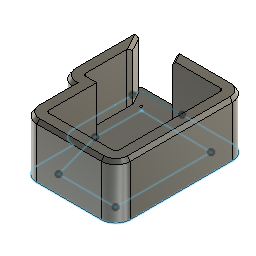
isopad-case-bigswitch v6 (Autodesk Fusion 360 design; units mm, degrees)
Autodesk Fusion 360 part; units mm, degrees
note: some values were not read from the file. Set by a fixed rule: which sketch regions a step uses.
(part 1 of 3)
sketch "isopad-Edge_Cuts" plane through (0, 0, 0) normal (0, 0, 1) x (1, 0, 0)
  line L0 (124.655, -116.632) -> (124.654, -116.632)
  line L1 (150.738, -76.6321) -> (150.718, -116.273)
  line L2 (125.094, -116.865) -> (125.093, -116.865)
  line L3 (150.127, -116.867) -> (150.124, -116.867)
  line L4 (150.128, -116.867) -> (150.127, -116.867)
  line L5 (124.654, -116.632) -> (124.653, -116.63)
  line L6 (150.242, -116.855) -> (150.24, -116.855)
  line L7 (150.718, -116.273) -> (150.718, -116.274)
  line L8 (150.707, -116.388) -> (150.706, -116.39)
  line L9 (124.653, -116.63) -> (124.652, -116.628)
  line L10 (124.652, -116.628) -> (124.605, -116.541)
  line L11 (150.723, -76.4882) -> (150.724, -76.4904)
  line L12 (150.718, -116.274) -> (150.707, -116.385)
  line L13 (150.738, -76.6246) -> (150.738, -76.625)
  line L14 (150.24, -116.855) -> (150.13, -116.867)
  line L15 (150.724, -76.4904) -> (150.724, -76.4927)
  line L16 (150.706, -116.39) -> (150.674, -116.496)
  line L17 (150.62, -116.599) -> (150.62, -116.599)
  line L18 (150.353, -116.82) -> (150.351, -116.821)
  line L19 (150.718, -116.274) -> (150.718, -116.274)
  line L20 (150.543, -116.693) -> (150.458, -116.764)
  line L21 (124.573, -116.437) -> (124.562, -116.338)
  line L22 (150.355, -116.82) -> (150.353, -116.82)
  line L23 (150.245, -116.854) -> (150.242, -116.855)
  line L24 (150.674, -116.496) -> (150.674, -116.497)
  line L25 (150.457, -116.764) -> (150.456, -116.765)
  line L26 (150.547, -116.69) -> (150.545, -116.691)
  line L27 (150.245, -116.854) -> (150.245, -116.854)
  line L28 (150.707, -116.386) -> (150.707, -116.388)
  line L29 (150.351, -116.821) -> (150.245, -116.854)
  line L30 (150.738, -76.625) -> (150.738, -76.6261)
  line L31 (150.707, -116.385) -> (150.707, -116.386)
  line L32 (150.356, -116.819) -> (150.355, -116.82)
  line L33 (150.62, -116.599) -> (150.618, -116.601)
  line L34 (150.13, -116.867) -> (150.129, -116.867)
  line L35 (150.456, -116.765) -> (150.454, -116.767)
  line L36 (150.454, -116.767) -> (150.356, -116.819)
  line L37 (150.618, -116.601) -> (150.617, -116.603)
  line L38 (150.123, -116.867) -> (125.094, -116.865)
  line L39 (150.545, -116.691) -> (150.543, -116.693)
  line L40 (150.672, -116.501) -> (150.62, -116.599)
  line L41 (150.129, -116.867) -> (150.128, -116.867)
  line L42 (150.124, -116.867) -> (150.124, -116.867)
  line L43 (150.547, -116.689) -> (150.547, -116.69)
  line L44 (150.673, -116.499) -> (150.672, -116.501)
  line L45 (150.458, -116.764) -> (150.457, -116.764)
  line L46 (150.674, -116.497) -> (150.673, -116.499)
  line L47 (150.124, -116.867) -> (150.123, -116.867)
  line L48 (150.738, -76.6308) -> (150.738, -76.6308)
  line L49 (150.738, -76.6272) -> (150.738, -76.6308)
  line L50 (124.562, -116.338) -> (124.562, -116.337)
  line L51 (150.738, -76.6261) -> (150.738, -76.6272)
  line L52 (150.723, -76.4879) -> (150.723, -76.4882)
  line L53 (124.718, -116.708) -> (124.655, -116.632)
  line L54 (150.738, -76.6319) -> (150.738, -76.6321)
  line L55 (150.738, -76.6308) -> (150.738, -76.6319)
  line L56 (150.724, -76.4927) -> (150.738, -76.6246)
  line L57 (150.617, -116.603) -> (150.547, -116.689)
  line L58 (124.605, -116.541) -> (124.605, -116.54)
  line L59 (124.894, -116.826) -> (124.894, -116.825)
  line L60 (122.341, -84.8701) -> (122.306, -84.865)
  line L61 (122.343, -84.8702) -> (122.341, -84.8701)
  line L62 (124.994, -116.855) -> (124.994, -116.855)
  line L63 (132.002, -76.3662) -> (132.03, -76.4168)
  line L64 (132.262, -75.917) -> (132.262, -75.917)
  line L65 (132.189, -75.9254) -> (132.191, -75.9249)
  line L66 (132.187, -75.9259) -> (132.189, -75.9254)
  line L67 (133.041, -78.8499) -> (133.086, -78.8196)
  line L68 (124.455, -97.412) -> (124.456, -97.4136)
  line L69 (119.228, -96.7752) -> (119.228, -96.7752)
  line L70 (124.994, -116.855) -> (124.991, -116.855)
  line L71 (122.301, -84.8638) -> (122.267, -84.8519)
  line L72 (119.228, -96.7744) -> (119.228, -96.7741)
  line L73 (124.991, -116.855) -> (124.989, -116.854)
  line L74 (122.306, -84.865) -> (122.305, -84.8649)
  line L75 (119.321, -97.074) -> (119.32, -97.0737)
  line L76 (122.263, -84.8498) -> (122.232, -84.8316)
  line L77 (150.035, -75.9271) -> (150.035, -75.9271)
  line L78 (124.573, -116.442) -> (124.573, -116.441)
  line L79 (124.798, -116.774) -> (124.721, -116.712)
  line L80 (124.453, -97.4102) -> (124.453, -97.4104)
  line L81 (122.305, -84.8649) -> (122.303, -84.8644)
  line L82 (122.267, -84.8519) -> (122.267, -84.8518)
  line L83 (124.573, -116.441) -> (124.573, -116.439)
  line L84 (122.303, -84.8644) -> (122.301, -84.8638)
  line L85 (124.284, -97.2983) -> (124.372, -97.3448)
  line L86 (133.068, -78.892) -> (133.068, -78.8922)
  line L87 (131.957, -76.3884) -> (131.957, -76.3881)
  line L88 (122.267, -84.8518) -> (122.265, -84.8508)
  line L89 (124.8, -116.776) -> (124.798, -116.774)
  line L90 (122.267, -84.8519) -> (122.267, -84.8519)
  line L91 (124.185, -97.2677) -> (124.28, -97.2964)
  line L92 (124.562, -116.336) -> (124.562, -116.333)
  line L93 (122.267, -84.8519) -> (122.267, -84.8519)
  line L94 (124.721, -116.712) -> (124.719, -116.71)
  line L95 (132.191, -75.9249) -> (132.251, -75.9173)
  line L96 (132.019, -76.0227) -> (132.021, -76.021)
  line L97 (131.98, -76.0726) -> (131.981, -76.0706)
  line L98 (131.979, -76.0744) -> (131.98, -76.0726)
  line L99 (131.928, -76.2567) -> (131.933, -76.1964)
  line L100 (132.019, -76.0229) -> (132.019, -76.0227)
  line L101 (124.802, -116.777) -> (124.8, -116.776)
  line L102 (124.604, -116.538) -> (124.603, -116.536)
  line L103 (132.254, -75.9171) -> (132.262, -75.917)
  line L104 (124.989, -116.854) -> (124.894, -116.826)
  line L105 (132.124, -75.9471) -> (132.125, -75.947)
  line L106 (132.263, -75.917) -> (132.263, -75.917)
  line L107 (131.933, -76.1938) -> (131.934, -76.1916)
  line L108 (131.95, -76.1333) -> (131.95, -76.133)
  line L109 (132.262, -75.917) -> (132.263, -75.917)
  line L110 (131.981, -76.0706) -> (132.019, -76.0229)
  line L111 (131.951, -76.1309) -> (131.952, -76.1288)
  line L112 (119.278, -86.6128) -> (119.278, -86.6128)
  line L113 (133.119, -78.8567) -> (133.118, -78.8582)
  line L114 (122.201, -84.8048) -> (122.201, -84.8046)
  line L115 (119.228, -86.6128) -> (119.226, -80.7208)
  line L116 (119.361, -97.044) -> (119.421, -97.1166)
  line L117 (133.195, -78.7636) -> (133.163, -78.8117)
  line L118 (119.233, -80.6444) -> (119.254, -80.5766)
  line L119 (122.175, -84.7712) -> (122.175, -84.7702)
  line L120 (122.201, -84.8046) -> (122.199, -84.8029)
  line L121 (124.802, -116.777) -> (124.802, -116.777)
  line L122 (119.611, -80.3346) -> (119.613, -80.3346)
  line L123 (124.562, -97.7901) -> (124.562, -97.7878)
  line L124 (122.265, -84.8508) -> (122.263, -84.8498)
  line L125 (119.387, -97.1536) -> (119.385, -97.152)
  line L126 (119.269, -96.9783) -> (119.239, -96.8835)
  line L127 (124.562, -97.7901) -> (124.562, -97.7901)
  line L128 (119.271, -96.9827) -> (119.271, -96.9824)
  line L129 (124.569, -97.5816) -> (124.57, -97.5837)
  line L130 (124.18, -97.2668) -> (124.18, -97.2668)
  line L131 (133.232, -78.6402) -> (133.232, -78.6424)
  line L132 (150.123, -116.817) -> (150.126, -116.817)
  line L133 (122.199, -84.8029) -> (122.198, -84.8012)
  line L134 (122.176, -84.7726) -> (122.176, -84.7723)
  line L135 (122.286, -84.8056) -> (122.315, -84.8159)
  line L136 (119.228, -96.7741) -> (119.228, -96.7737)
  line L137 (124.346, -97.3878) -> (124.263, -97.3436)
  line L138 (119.891, -80.5315) -> (119.849, -80.481)
  line L139 (150.233, -116.806) -> (150.334, -116.774)
  line L140 (124.562, -116.338) -> (124.562, -116.338)
  line L141 (119.228, -96.7787) -> (119.228, -96.7776)
  line L142 (124.562, -116.333) -> (124.562, -116.333)
  line L143 (132.072, -75.977) -> (132.124, -75.9471)
  line L144 (122.231, -84.8314) -> (122.23, -84.83)
  line L145 (124.562, -116.337) -> (124.562, -116.336)
  line L146 (119.316, -96.9611) -> (119.361, -97.044)
  line L147 (119.686, -80.3415) -> (119.688, -80.3419)
  line L148 (124.521, -97.4922) -> (124.522, -97.494)
  line L149 (124.562, -116.333) -> (124.562, -97.7901)
  line L150 (119.228, -96.7798) -> (119.228, -96.7787)
  line L151 (119.466, -97.2178) -> (119.464, -97.2165)
  line L152 (124.552, -97.6929) -> (124.524, -97.6029)
  line L153 (119.533, -80.343) -> (119.533, -80.3429)
  line L154 (124.573, -116.439) -> (124.573, -116.437)
  line L155 (122.228, -84.8287) -> (122.201, -84.8048)
  line L156 (119.964, -80.5589) -> (119.964, -80.5591)
  line L157 (119.289, -80.5094) -> (119.29, -80.5075)
  line L158 (124.721, -116.712) -> (124.721, -116.712)
  line L159 (124.569, -97.5813) -> (124.569, -97.5816)
  line L160 (150.16, -75.9896) -> (150.032, -75.977)
  line L161 (122.236, -84.7692) -> (122.259, -84.7898)
  line L162 (124.612, -97.7853) -> (124.612, -97.7864)
  line L163 (131.936, -76.3264) -> (131.936, -76.3261)
  line L164 (122.198, -84.8012) -> (122.176, -84.7726)
  line L165 (122.215, -84.7397) -> (122.217, -84.7437)
  line L166 (122.23, -84.83) -> (122.228, -84.8287)
  line L167 (122.232, -84.8316) -> (122.231, -84.8314)
  line L168 (133.171, -78.5331) -> (133.151, -78.4836)
  line L169 (122.425, -84.8575) -> (122.423, -84.8582)
  line L170 (122.346, -84.8703) -> (122.346, -84.8703)
  line L171 (119.461, -80.3658) -> (119.461, -80.3657)
  line L172 (124.601, -97.6852) -> (124.612, -97.7838)
  line L173 (133.22, -78.5208) -> (133.231, -78.5773)
  line L174 (133.197, -78.7596) -> (133.196, -78.7616)
  line L175 (131.979, -76.0748) -> (131.979, -76.0747)
  line L176 (132.022, -76.0194) -> (132.068, -75.9798)
  line L177 (132.068, -75.9796) -> (132.07, -75.9783)
  line L178 (122.176, -84.7723) -> (122.175, -84.7712)
  line L179 (122.346, -84.8203) -> (122.377, -84.8187)
  line L180 (122.407, -84.8111) -> (122.436, -84.7972)
  line L181 (124.562, -97.7878) -> (124.552, -97.6929)
  line L182 (122.175, -84.7702) -> (122.172, -84.7653)
  line L183 (119.823, -80.3965) -> (119.823, -80.3967)
  line L184 (131.978, -76.2581) -> (131.985, -76.3133)
  line L185 (119.233, -80.6492) -> (119.233, -80.6488)
  line L186 (119.882, -80.4435) -> (119.882, -80.4435)
  line L187 (119.931, -80.5011) -> (119.931, -80.5014)
  line L188 (124.601, -97.6808) -> (124.601, -97.683)
  line L189 (119.292, -80.5056) -> (119.336, -80.4508)
  line L190 (124.524, -97.6029) -> (124.479, -97.52)
  line L191 (119.921, -80.5841) -> (119.891, -80.5315)
  line L192 (119.464, -97.2165) -> (119.387, -97.1538)
  line L193 (124.479, -97.52) -> (124.419, -97.4474)
  line L194 (119.884, -80.4454) -> (119.886, -80.4469)
  line L195 (133.12, -78.8565) -> (133.12, -78.8565)
  line L196 (119.931, -80.5014) -> (119.933, -80.5032)
  line L197 (122.172, -84.7653) -> (122.172, -84.7649)
  line L198 (150.126, -116.817) -> (150.233, -116.806)
  line L199 (122.458, -84.8421) -> (122.426, -84.8574)
  line L200 (119.254, -80.5766) -> (119.254, -80.5763)
  line L201 (133.086, -78.8196) -> (133.123, -78.7821)
  line L202 (150.428, -116.724) -> (150.51, -116.656)
  line L203 (131.933, -76.196) -> (131.933, -76.1938)
  line L204 (131.955, -76.384) -> (131.936, -76.3264)
  line L205 (119.535, -80.3425) -> (119.537, -80.3421)
  line L206 (119.762, -97.257) -> (124.08, -97.257)
  line L207 (133.197, -78.7593) -> (133.197, -78.7596)
  line L208 (133.197, -78.4646) -> (133.197, -78.4649)
  line L209 (119.886, -80.4469) -> (119.931, -80.5011)
  line L210 (124.419, -97.4474) -> (124.346, -97.3878)
  line L211 (122.172, -84.7649) -> (119.921, -80.5841)
  line L212 (124.28, -97.2964) -> (124.28, -97.2965)
  line L213 (124.612, -97.7888) -> (124.612, -116.332)
  line L214 (150.688, -76.6321) -> (150.688, -76.6286)
  line L215 (133.232, -78.6447) -> (133.22, -78.7012)
  line L216 (124.828, -116.734) -> (124.911, -116.778)
  line L217 (119.34, -80.4473) -> (119.394, -80.4022)
  line L218 (119.608, -80.3347) -> (119.608, -80.3346)
  line L219 (124.601, -97.683) -> (124.601, -97.6852)
  line L220 (119.537, -80.3421) -> (119.608, -80.3347)
  line L221 (124.612, -97.7864) -> (124.612, -97.7887)
  line L222 (119.226, -80.7196) -> (119.226, -80.7196)
  line L223 (150.688, -76.6286) -> (150.675, -76.5003)
  line L224 (150.576, -76.2658) -> (150.494, -76.1673)
  line L225 (124.605, -116.54) -> (124.604, -116.538)
  line L226 (133.163, -78.8117) -> (133.163, -78.812)
  line L227 (133.163, -78.812) -> (133.162, -78.8137)
  line L228 (132.263, -75.917) -> (150.034, -75.927)
  line L229 (132.251, -75.9173) -> (132.253, -75.9173)
  line L230 (150.032, -75.977) -> (132.263, -75.967)
  line L231 (119.684, -80.3411) -> (119.686, -80.3415)
  line L232 (119.397, -80.4008) -> (119.398, -80.3995)
  line L233 (133.152, -78.7381) -> (133.172, -78.6893)
  line L234 (119.758, -80.3629) -> (119.76, -80.3637)
  line L235 (150.675, -76.5003) -> (150.637, -76.3782)
  line L236 (119.688, -80.3419) -> (119.756, -80.3619)
  line L237 (119.228, -96.7776) -> (119.228, -96.7752)
  line L238 (150.494, -76.1673) -> (150.395, -76.0865)
  line L239 (119.228, -96.7802) -> (119.228, -96.7798)
  line L240 (119.278, -86.6128) -> (119.278, -96.7739)
  line L241 (150.123, -116.817) -> (150.123, -116.817)
  line L242 (119.398, -80.3995) -> (119.461, -80.3658)
  line L243 (119.465, -80.364) -> (119.533, -80.343)
  line L244 (132.256, -75.9671) -> (132.2, -75.9742)
  line L245 (119.556, -97.2657) -> (119.468, -97.2192)
  line L246 (150.627, -116.48) -> (150.658, -116.378)
  line L247 (133.219, -78.5165) -> (133.219, -78.5187)
  line L248 (119.394, -80.4022) -> (119.395, -80.402)
  line L249 (124.57, -97.5837) -> (124.571, -97.5857)
  line L250 (119.882, -80.4435) -> (119.882, -80.4435)
  line L251 (133.172, -78.6893) -> (133.182, -78.6375)
  line L252 (124.612, -97.7842) -> (124.612, -97.7853)
  line L253 (119.558, -97.2666) -> (119.556, -97.2657)
  line L254 (122.423, -84.8582) -> (122.421, -84.859)
  line L255 (122.386, -84.8679) -> (122.384, -84.8682)
  line L256 (119.461, -80.3657) -> (119.463, -80.3648)
  line L257 (119.233, -80.6488) -> (119.233, -80.6466)
  line L258 (124.376, -97.3475) -> (124.453, -97.4102)
  line L259 (119.233, -80.6466) -> (119.233, -80.6444)
  line L260 (150.577, -116.574) -> (150.627, -116.48)
  line L261 (133.123, -78.7821) -> (133.152, -78.7381)
  line L262 (119.226, -80.7196) -> (119.233, -80.6492)
  line L263 (124.456, -97.4136) -> (124.519, -97.49)
  line L264 (119.301, -80.5934) -> (119.282, -80.6565)
  line L265 (133.219, -78.5187) -> (133.22, -78.5208)
  line L266 (119.276, -80.7232) -> (119.278, -86.6128)
  line L267 (133.231, -78.5773) -> (133.231, -78.5777)
  line L268 (124.522, -97.494) -> (124.569, -97.5813)
  line L269 (119.56, -97.2676) -> (119.56, -97.2675)
  line L270 (119.655, -97.2963) -> (119.56, -97.2676)
  line L271 (119.226, -80.7208) -> (119.226, -80.7196)
  line L272 (124.65, -116.519) -> (124.695, -116.602)
  line L273 (119.56, -97.2675) -> (119.558, -97.2666)
  line L274 (119.338, -80.4489) -> (119.34, -80.4473)
  line L275 (119.282, -80.6565) -> (119.276, -80.7232)
  line L276 (131.997, -76.1491) -> (131.982, -76.2027)
  line L277 (122.259, -84.7898) -> (122.286, -84.8056)
  line L278 (119.468, -97.2192) -> (119.468, -97.219)
  line L279 (124.612, -97.7887) -> (124.612, -97.7888)
  line L280 (133.182, -78.5848) -> (133.171, -78.5331)
  line L281 (119.683, -80.341) -> (119.684, -80.3411)
  line L282 (119.494, -97.1762) -> (119.577, -97.2204)
  line L283 (119.319, -97.0718) -> (119.318, -97.07)
  line L284 (150.51, -116.656) -> (150.577, -116.574)
  line L285 (124.52, -97.4903) -> (124.521, -97.4922)
  line L286 (119.759, -97.3069) -> (119.66, -97.2972)
  line L287 (119.424, -80.4423) -> (119.374, -80.4843)
  line L288 (119.577, -97.2204) -> (119.667, -97.2477)
  line L289 (119.385, -97.152) -> (119.384, -97.1504)
  line L290 (119.66, -97.2972) -> (119.657, -97.2967)
  line L291 (124.372, -97.345) -> (124.374, -97.3462)
  line L292 (124.183, -97.2673) -> (124.185, -97.2677)
  line L293 (119.387, -97.1538) -> (119.387, -97.1536)
  line L294 (131.936, -76.3261) -> (131.936, -76.3239)
  line L295 (119.374, -80.4843) -> (119.332, -80.5353)
  line L296 (124.282, -97.2974) -> (124.284, -97.2983)
  line L297 (119.278, -96.7762) -> (119.288, -96.8711)
  line L298 (119.827, -80.3992) -> (119.882, -80.4435)
  line L299 (124.18, -97.2668) -> (124.183, -97.2673)
  line L300 (119.384, -97.1504) -> (119.321, -97.074)
  line L301 (122.217, -84.7437) -> (122.236, -84.7692)
  line L302 (119.278, -96.7739) -> (119.278, -96.7762)
  line L303 (133.232, -78.5822) -> (133.232, -78.6398)
  line L304 (124.612, -97.7838) -> (124.612, -97.7842)
  line L305 (124.519, -97.49) -> (124.52, -97.4903)
  line L306 (119.288, -96.8711) -> (119.316, -96.9611)
  line L307 (119.228, -96.7737) -> (119.228, -86.6128)
  line L308 (119.318, -97.07) -> (119.271, -96.9827)
  line L309 (124.374, -97.3462) -> (124.376, -97.3475)
  line L310 (150.334, -116.774) -> (150.428, -116.724)
  line L311 (119.228, -96.7752) -> (119.228, -96.7744)
  line L312 (119.657, -97.2967) -> (119.655, -97.2963)
  line L313 (150.395, -76.0865) -> (150.283, -76.0265)
  line L314 (133.22, -78.7012) -> (133.22, -78.7016)
  line L315 (119.545, -80.3915) -> (119.482, -80.411)
  line L316 (119.934, -80.5049) -> (119.964, -80.5589)
  line L317 (119.533, -80.3429) -> (119.535, -80.3425)
  line L318 (124.28, -97.2965) -> (124.282, -97.2974)
  line L319 (119.76, -97.307) -> (119.759, -97.3069)
  line L320 (119.676, -80.3906) -> (119.611, -80.3846)
  line L321 (124.08, -97.257) -> (124.081, -97.2571)
  line L322 (133.196, -78.7616) -> (133.195, -78.7636)
  line L323 (124.571, -97.5857) -> (124.601, -97.6805)
  line L324 (119.336, -80.4508) -> (119.337, -80.4505)
  line L325 (119.613, -80.3346) -> (119.683, -80.341)
  line L326 (133.231, -78.5777) -> (133.232, -78.5799)
  line L327 (133.219, -78.5162) -> (133.219, -78.5165)
  line L328 (119.239, -96.8832) -> (119.239, -96.881)
  line L329 (132.263, -75.917) -> (132.263, -75.917)
  line L330 (150.034, -75.927) -> (150.035, -75.9271)
  line L331 (122.377, -84.8187) -> (122.407, -84.8111)
  line L332 (119.482, -80.411) -> (119.424, -80.4423)
  line L333 (119.608, -80.3346) -> (119.611, -80.3346)
  line L334 (119.228, -86.6128) -> (119.228, -86.6128)
  line L335 (124.263, -97.3436) -> (124.173, -97.3163)
  line L336 (119.239, -96.881) -> (119.239, -96.8788)
  line L337 (119.849, -80.481) -> (119.798, -80.4397)
  line L338 (119.66, -97.2972) -> (119.66, -97.2972)
  line L339 (119.332, -80.5353) -> (119.301, -80.5934)
  line L340 (124.453, -97.4104) -> (124.455, -97.412)
  line L341 (119.468, -97.219) -> (119.466, -97.2178)
  line L342 (119.32, -97.0737) -> (119.319, -97.0718)
  line L343 (124.601, -97.6805) -> (124.601, -97.6808)
  line L344 (119.239, -96.8788) -> (119.228, -96.7802)
  line L345 (133.232, -78.6398) -> (133.232, -78.6402)
  line L346 (124.081, -97.2571) -> (124.18, -97.2668)
  line L347 (119.611, -80.3846) -> (119.545, -80.3915)
  line L348 (119.739, -80.4092) -> (119.676, -80.3906)
  line L349 (133.182, -78.6375) -> (133.182, -78.5848)
  line L350 (119.463, -80.3648) -> (119.465, -80.364)
  line L351 (124.755, -116.675) -> (124.828, -116.734)
  line L352 (124.372, -97.3448) -> (124.372, -97.345)
  line L353 (124.081, -97.2571) -> (124.081, -97.2571)
  line L354 (119.964, -80.5591) -> (122.215, -84.7397)
  line L355 (119.759, -97.3069) -> (119.759, -97.3069)
  line L356 (119.271, -96.9824) -> (119.27, -96.9803)
  line L357 (119.667, -97.2477) -> (119.762, -97.257)
  line L358 (119.27, -96.9803) -> (119.269, -96.9783)
  line L359 (124.078, -97.307) -> (119.76, -97.307)
  line L360 (119.239, -96.8835) -> (119.239, -96.8832)
  line L361 (119.421, -97.1166) -> (119.494, -97.1762)
  line L362 (133.12, -78.8565) -> (133.12, -78.8565)
  line L363 (119.29, -80.5075) -> (119.292, -80.5056)
  line L364 (150.283, -76.0265) -> (150.16, -75.9896)
  line L365 (150.637, -76.3782) -> (150.576, -76.2658)
  line L366 (119.756, -80.362) -> (119.758, -80.3629)
  line L367 (131.936, -76.3239) -> (131.935, -76.3217)
  line L368 (133.196, -78.4612) -> (133.197, -78.4646)
  line L369 (122.421, -84.859) -> (122.386, -84.8678)
  line L370 (122.386, -84.8678) -> (122.386, -84.8679)
  line L371 (131.95, -76.133) -> (131.951, -76.1309)
  line L372 (124.173, -97.3163) -> (124.078, -97.307)
  line L373 (131.957, -76.3881) -> (131.956, -76.386)
  line L374 (133.197, -78.4649) -> (133.219, -78.5162)
  line L375 (150.668, -116.271) -> (150.688, -76.6321)
  line L376 (119.798, -80.4397) -> (119.739, -80.4092)
  line L377 (133.232, -78.5799) -> (133.232, -78.5822)
  line L378 (125.096, -116.815) -> (150.123, -116.817)
  line L379 (133.232, -78.6424) -> (133.232, -78.6447)
  line L380 (125.001, -116.806) -> (125.096, -116.815)
  line L381 (119.395, -80.402) -> (119.397, -80.4008)
  line L382 (119.337, -80.4505) -> (119.338, -80.4489)
  line L383 (119.256, -80.5721) -> (119.289, -80.5097)
  line L384 (119.255, -80.5742) -> (119.256, -80.5721)
  line L385 (122.426, -84.8574) -> (122.425, -84.8575)
  line L386 (122.459, -84.8418) -> (122.458, -84.8421)
  line L387 (124.911, -116.778) -> (125.001, -116.806)
  line L388 (119.289, -80.5097) -> (119.289, -80.5094)
  line L389 (124.612, -116.332) -> (124.612, -116.334)
  line L390 (122.315, -84.8159) -> (122.346, -84.8203)
  line L391 (150.658, -116.378) -> (150.668, -116.271)
  line L392 (119.933, -80.5032) -> (119.934, -80.5049)
  line L393 (119.254, -80.5763) -> (119.255, -80.5742)
  line L394 (131.952, -76.1288) -> (131.979, -76.0748)
  line L395 (124.612, -116.334) -> (124.622, -116.429)
  line L396 (124.622, -116.429) -> (124.65, -116.519)
  line L397 (124.695, -116.602) -> (124.755, -116.675)
  line L398 (131.979, -76.0747) -> (131.979, -76.0747)
  line L399 (133.067, -78.8927) -> (133.066, -78.8933)
  line L400 (132.057, -76.0556) -> (132.022, -76.0995)
  line L401 (132.021, -76.021) -> (132.022, -76.0194)
  line L402 (133.162, -78.8137) -> (133.16, -78.8155)
  line L403 (133.066, -78.8933) -> (133.065, -78.8939)
  line L404 (131.935, -76.3217) -> (131.928, -76.2616)
  line L405 (131.986, -76.4404) -> (131.986, -76.4403)
  line L406 (131.933, -76.1964) -> (131.933, -76.196)
  line L407 (133.22, -78.7038) -> (133.219, -78.7059)
  line L408 (131.928, -76.2616) -> (131.928, -76.2612)
  line L409 (150.168, -75.9401) -> (150.168, -75.9401)
  line L410 (150.035, -75.9271) -> (150.168, -75.9401)
  line L411 (122.384, -84.8682) -> (122.382, -84.8685)
  line L412 (150.168, -75.9401) -> (150.168, -75.9401)
  line L413 (133.118, -78.8582) -> (133.116, -78.8596)
  line L414 (122.346, -84.8703) -> (122.346, -84.8704)
  line L415 (132.186, -75.926) -> (132.187, -75.9259)
  line L416 (132.129, -75.9451) -> (132.186, -75.926)
  line L417 (132.253, -75.9173) -> (132.254, -75.9171)
  line L418 (133.065, -78.8939) -> (122.459, -84.8418)
  line L419 (133.16, -78.8155) -> (133.12, -78.8565)
  line L420 (131.956, -76.386) -> (131.955, -76.384)
  line L421 (132.07, -75.9783) -> (132.072, -75.977)
  line L422 (133.068, -78.8922) -> (133.067, -78.8927)
  line L423 (133.116, -78.8596) -> (133.068, -78.892)
  line L424 (122.346, -84.8704) -> (122.343, -84.8702)
  line L425 (131.986, -76.4403) -> (131.957, -76.3884)
  line L426 (133.219, -78.7059) -> (133.197, -78.7593)
  line L427 (132.127, -75.9461) -> (132.129, -75.9451)
  line L428 (131.979, -76.0747) -> (131.979, -76.0744)
  line L429 (132.186, -75.926) -> (132.186, -75.926)
  line L430 (132.068, -75.9798) -> (132.068, -75.9796)
  line L431 (131.928, -76.259) -> (131.928, -76.2567)
  line L432 (122.382, -84.8685) -> (122.346, -84.8703)
  line L433 (131.982, -76.2027) -> (131.978, -76.2581)
  line L434 (133.151, -78.4836) -> (131.986, -76.4404)
  line L435 (122.436, -84.7972) -> (133.041, -78.8499)
  line L436 (119.882, -80.4435) -> (119.883, -80.4437)
  line L437 (132.022, -76.0995) -> (131.997, -76.1491)
  line L438 (119.823, -80.3967) -> (119.825, -80.398)
  line L439 (132.263, -75.967) -> (132.256, -75.9671)
  line L440 (132.099, -76.0193) -> (132.057, -76.0556)
  line L441 (133.22, -78.7016) -> (133.22, -78.7038)
  line L442 (132.03, -76.4168) -> (133.196, -78.4612)
  line L443 (132.2, -75.9742) -> (132.147, -75.9918)
  line L444 (119.756, -80.3619) -> (119.756, -80.362)
  line L445 (133.12, -78.8565) -> (133.119, -78.8567)
  line L446 (119.883, -80.4437) -> (119.884, -80.4454)
  line L447 (119.76, -80.3637) -> (119.823, -80.3965)
  line L448 (132.147, -75.9918) -> (132.099, -76.0193)
  line L449 (124.719, -116.71) -> (124.718, -116.708)
  line L450 (131.928, -76.2612) -> (131.928, -76.259)
  line L451 (119.825, -80.398) -> (119.827, -80.3992)
  line L452 (132.251, -75.9173) -> (132.251, -75.9173)
  line L453 (131.985, -76.3133) -> (132.002, -76.3662)
  line L454 (131.934, -76.1916) -> (131.95, -76.1333)
  line L455 (132.125, -75.947) -> (132.127, -75.9461)
  line L456 (150.421, -76.0437) -> (150.423, -76.045)
  line L457 (150.528, -76.1301) -> (150.528, -76.1301)
  line L458 (150.299, -75.9794) -> (150.299, -75.9794)
  line L459 (150.682, -76.3566) -> (150.682, -76.3569)
  line L460 (150.299, -75.9794) -> (150.3, -75.9795)
  line L461 (150.684, -76.3611) -> (150.723, -76.4879)
  line L462 (150.423, -76.045) -> (150.425, -76.0462)
  line L463 (150.421, -76.0435) -> (150.421, -76.0435)
  line L464 (150.172, -75.941) -> (150.299, -75.9794)
  line L465 (150.619, -76.2399) -> (150.682, -76.3566)
  line L466 (150.53, -76.1319) -> (150.531, -76.1336)
  line L467 (150.3, -75.9795) -> (150.302, -75.9804)
  line L468 (150.528, -76.1301) -> (150.528, -76.1301)
  line L469 (150.302, -75.9804) -> (150.304, -75.9812)
  line L470 (150.528, -76.1301) -> (150.528, -76.1303)
  line L471 (150.421, -76.0435) -> (150.421, -76.0437)
  line L472 (150.616, -76.2361) -> (150.617, -76.238)
  line L473 (150.616, -76.2358) -> (150.616, -76.2361)
  line L474 (150.683, -76.359) -> (150.684, -76.3611)
  line L475 (150.682, -76.3569) -> (150.683, -76.359)
  line L476 (150.617, -76.238) -> (150.619, -76.2399)
  line L477 (150.425, -76.0462) -> (150.528, -76.1301)
  line L478 (150.531, -76.1336) -> (150.616, -76.2358)
  line L479 (124.892, -116.825) -> (124.89, -116.824)
  line L480 (150.304, -75.9812) -> (150.421, -76.0435)
  line L481 (150.421, -76.0435) -> (150.421, -76.0435)
  line L482 (124.89, -116.824) -> (124.802, -116.777)
  line L483 (124.894, -116.825) -> (124.892, -116.825)
  line L484 (150.528, -76.1303) -> (150.53, -76.1319)
  line L485 (150.168, -75.9401) -> (150.17, -75.9406)
  line L486 (150.17, -75.9406) -> (150.172, -75.941)
  line L487 (124.603, -116.536) -> (124.573, -116.442)
  line L488 (125.093, -116.865) -> (124.994, -116.855)
  line L489 (125.093, -116.865) -> (125.093, -116.865)
  line L490 (138.121, -85.0559) -> (138.264, -84.96)
  line L491 (138.264, -84.96) -> (138.424, -84.8939)
  line L492 (138.424, -84.8939) -> (138.593, -84.8603)
  line L493 (145.099, -104.104) -> (145.197, -104.202)
  line L494 (145.197, -104.202) -> (145.273, -104.316)
  line L495 (145.353, -104.717) -> (145.326, -104.852)
  line L496 (145.326, -104.852) -> (145.273, -104.98)
  line L497 (145.273, -104.98) -> (145.197, -105.094)
  line L498 (138.593, -84.8603) -> (138.765, -84.8603)
  line L499 (138.765, -84.8603) -> (138.935, -84.8939)
  line L500 (129.741, -82.4107) -> (130.103, -82.561)
  line L501 (145.273, -104.316) -> (145.326, -104.444)
  line L502 (145.326, -104.444) -> (145.353, -104.579)
  line L503 (145.353, -104.579) -> (145.353, -104.717)
  line L504 (132.643, -96.9881) -> (132.817, -96.9535)
  line L505 (132.817, -96.9535) -> (132.994, -96.9535)
  line L506 (132.994, -96.9535) -> (133.168, -96.9881)
  line L507 (128.276, -96.9133) -> (128.436, -96.9794)
  line L508 (137.733, -104.579) -> (137.733, -104.717)
  line L509 (144.536, -94.1203) -> (144.602, -94.2798)
  line L510 (144.602, -94.2798) -> (144.635, -94.4491)
  line L511 (144.635, -94.4491) -> (144.635, -94.6217)
  line L512 (132.206, -97.2798) -> (132.332, -97.1544)
  line L513 (132.332, -97.1544) -> (132.479, -97.0559)
  line L514 (132.479, -97.0559) -> (132.643, -96.9881)
  line L515 (136.587, -105.192) -> (136.489, -105.094)
  line L516 (132.005, -97.9421) -> (132.005, -97.7649)
  line L517 (136.734, -100.788) -> (136.856, -100.666)
  line L518 (136.856, -100.666) -> (137, -100.571)
  line L519 (132.005, -97.7649) -> (132.04, -97.591)
  line L520 (132.04, -97.591) -> (132.108, -97.4272)
  line L521 (132.108, -97.4272) -> (132.206, -97.2798)
  line L522 (145.099, -105.192) -> (144.985, -105.268)
  line L523 (144.985, -105.268) -> (144.857, -105.321)
  line L524 (144.857, -105.321) -> (144.722, -105.348)
  line L525 (128.448, -99.7001) -> (128.514, -99.5406)
  line L526 (136.851, -84.2175) -> (136.728, -84.0955)
  line L527 (136.728, -84.0955) -> (136.633, -83.9519)
  line L528 (136.633, -83.9519) -> (136.566, -83.7925)
  line L529 (136.36, -104.444) -> (136.413, -104.316)
  line L530 (136.413, -104.316) -> (136.489, -104.202)
  line L531 (136.489, -104.202) -> (136.587, -104.104)
  line L532 (137.323, -82.6606) -> (137.495, -82.6606)
  line L533 (137.495, -82.6606) -> (137.665, -82.6942)
  line L534 (136.395, -80.4945) -> (136.554, -80.5606)
  line L535 (137.733, -104.717) -> (137.706, -104.852)
  line L536 (137.706, -104.852) -> (137.653, -104.98)
  line L537 (137.653, -104.98) -> (137.577, -105.094)
  line L538 (142.575, -93.212) -> (142.403, -93.212)
  line L539 (142.403, -93.212) -> (142.234, -93.1783)
  line L540 (142.234, -93.1783) -> (142.074, -93.1122)
  line L541 (142.074, -93.1122) -> (141.931, -93.0163)
  line L542 (141.931, -93.0163) -> (141.808, -92.8943)
  line L543 (136.566, -83.2812) -> (136.633, -83.1218)
  line L544 (136.633, -83.1218) -> (136.728, -82.9782)
  line L545 (136.728, -82.9782) -> (136.851, -82.8562)
  line L546 (136.587, -104.104) -> (136.701, -104.028)
  line L547 (136.701, -104.028) -> (136.829, -103.975)
  line L548 (136.829, -103.975) -> (136.964, -103.948)
  line L549 (135.263, -81.4235) -> (135.263, -81.2508)
  line L550 (135.263, -81.2508) -> (135.296, -81.0815)
  line L551 (135.296, -81.0815) -> (135.363, -80.9221)
  line L552 (136.554, -80.5606) -> (136.698, -80.6565)
  line L553 (136.698, -80.6565) -> (136.82, -80.7785)
  line L554 (136.82, -80.7785) -> (136.916, -80.9221)
  line L555 (139.094, -86.5131) -> (138.935, -86.5792)
  line L556 (138.935, -86.5792) -> (138.765, -86.6129)
  line L557 (138.765, -86.6129) -> (138.593, -86.6129)
  line L558 (149.532, -116.473) -> (149.213, -116.605)
  line L559 (150.453, -114.75) -> (150.453, -115.094)
  line L560 (136.82, -81.8958) -> (136.698, -82.0178)
  line L561 (136.698, -82.0178) -> (136.554, -82.1137)
  line L562 (136.554, -82.1137) -> (136.395, -82.1798)
  line L563 (142.904, -93.1122) -> (142.745, -93.1783)
  line L564 (142.745, -93.1783) -> (142.575, -93.212)
  line L565 (136.333, -104.717) -> (136.333, -104.579)
  line L566 (136.333, -104.579) -> (136.36, -104.444)
  line L567 (137, -100.571) -> (137.159, -100.505)
  line L568 (137.159, -100.505) -> (137.328, -100.471)
  line L569 (137.328, -100.471) -> (137.5, -100.471)
  line L570 (137.5, -100.471) -> (137.669, -100.505)
  line L571 (137.102, -103.948) -> (137.237, -103.975)
  line L572 (144.857, -103.975) -> (144.985, -104.028)
  line L573 (144.985, -104.028) -> (145.099, -104.104)
  line L574 (130.103, -82.561) -> (130.43, -82.7792)
  line L575 (130.43, -82.7792) -> (130.708, -83.057)
  line L576 (130.708, -83.057) -> (130.926, -83.3835)
  line L577 (137.365, -105.268) -> (137.237, -105.321)
  line L578 (137.237, -105.321) -> (137.102, -105.348)
  line L579 (137.102, -105.348) -> (136.964, -105.348)
  line L580 (145.197, -105.094) -> (145.099, -105.192)
  line L581 (137.577, -105.094) -> (137.479, -105.192)
  line L582 (137.479, -105.192) -> (137.365, -105.268)
  line L583 (136.964, -103.948) -> (137.102, -103.948)
  line L584 (136.489, -105.094) -> (136.413, -104.98)
  line L585 (136.413, -104.98) -> (136.36, -104.852)
  line L586 (136.36, -104.852) -> (136.333, -104.717)
  line L587 (148.753, -102.458) -> (148.925, -102.458)
  line L588 (148.925, -102.458) -> (149.095, -102.492)
  line L589 (130.816, -101.313) -> (130.976, -101.379)
  line L590 (130.976, -101.379) -> (131.119, -101.475)
  line L591 (136.964, -105.348) -> (136.829, -105.321)
  line L592 (136.829, -105.321) -> (136.701, -105.268)
  line L593 (136.701, -105.268) -> (136.587, -105.192)
  line L594 (135.363, -80.9221) -> (135.458, -80.7785)
  line L595 (135.458, -80.7785) -> (135.581, -80.6565)
  line L596 (135.581, -80.6565) -> (135.724, -80.5606)
  line L597 (130.926, -83.3835) -> (131.076, -83.7464)
  line L598 (131.076, -83.7464) -> (131.153, -84.1316)
  line L599 (131.153, -84.1316) -> (131.153, -84.5244)
  line L600 (136.566, -83.7925) -> (136.533, -83.6232)
  line L601 (136.533, -83.6232) -> (136.533, -83.4505)
  line L602 (136.533, -83.4505) -> (136.566, -83.2812)
  line L603 (136.851, -82.8562) -> (136.994, -82.7603)
  line L604 (136.994, -82.7603) -> (137.154, -82.6942)
  line L605 (137.154, -82.6942) -> (137.323, -82.6606)
  line L606 (131.153, -84.5244) -> (131.076, -84.9096)
  line L607 (131.076, -84.9096) -> (130.926, -85.2725)
  line L608 (130.926, -85.2725) -> (130.708, -85.599)
  line L609 (136.916, -80.9221) -> (136.982, -81.0815)
  line L610 (136.982, -81.0815) -> (137.015, -81.2508)
  line L611 (137.015, -81.2508) -> (137.015, -81.4235)
  line L612 (136.395, -82.1798) -> (136.225, -82.2135)
  line L613 (136.225, -82.2135) -> (136.053, -82.2135)
  line L614 (136.053, -82.2135) -> (135.884, -82.1798)
  line L615 (139.456, -86.1516) -> (139.36, -86.2952)
  line L616 (139.36, -86.2952) -> (139.238, -86.4172)
  line L617 (139.238, -86.4172) -> (139.094, -86.5131)
  line L618 (137.015, -81.4235) -> (136.982, -81.5928)
  line L619 (136.982, -81.5928) -> (136.916, -81.7522)
  line L620 (136.916, -81.7522) -> (136.82, -81.8958)
  line L621 (135.458, -81.8958) -> (135.363, -81.7522)
  line L622 (135.363, -81.7522) -> (135.296, -81.5928)
  line L623 (135.296, -81.5928) -> (135.263, -81.4235)
  line L624 (138.593, -86.6129) -> (138.424, -86.5792)
  line L625 (138.424, -86.5792) -> (138.264, -86.5131)
  line L626 (138.264, -86.5131) -> (138.121, -86.4172)
  line L627 (137.824, -84.3134) -> (137.665, -84.3795)
  line L628 (137.665, -84.3795) -> (137.495, -84.4132)
  line L629 (137.495, -84.4132) -> (137.323, -84.4132)
  line L630 (138.121, -86.4172) -> (137.998, -86.2952)
  line L631 (137.998, -86.2952) -> (137.903, -86.1516)
  line L632 (137.903, -86.1516) -> (137.836, -85.9922)
  line L633 (137.323, -84.4132) -> (137.154, -84.3795)
  line L634 (137.154, -84.3795) -> (136.994, -84.3134)
  line L635 (136.994, -84.3134) -> (136.851, -84.2175)
  line L636 (137.836, -85.481) -> (137.903, -85.3215)
  line L637 (137.903, -85.3215) -> (137.998, -85.178)
  line L638 (137.998, -85.178) -> (138.121, -85.0559)
  line L639 (135.884, -82.1798) -> (135.724, -82.1137)
  line L640 (135.724, -82.1137) -> (135.581, -82.0178)
  line L641 (135.581, -82.0178) -> (135.458, -81.8958)
  line L642 (137.836, -85.9922) -> (137.803, -85.8229)
  line L643 (137.803, -85.8229) -> (137.803, -85.6503)
  line L644 (137.803, -85.6503) -> (137.836, -85.481)
  line L645 (135.712, -79.3931) -> (135.646, -79.5525)
  line L646 (135.646, -79.5525) -> (135.55, -79.6961)
  line L647 (135.55, -79.6961) -> (135.428, -79.8181)
  line L648 (140.443, -89.7209) -> (140.538, -89.5774)
  line L649 (140.538, -89.5774) -> (140.661, -89.4553)
  line L650 (140.661, -89.4553) -> (140.804, -89.3594)
  line L651 (124.638, -93.6122) -> (124.605, -93.4429)
  line L652 (124.605, -93.4429) -> (124.605, -93.2703)
  line L653 (134.955, -80.0137) -> (134.783, -80.0137)
  line L654 (134.783, -80.0137) -> (134.614, -79.9801)
  line L655 (134.614, -79.9801) -> (134.454, -79.914)
  line L656 (122.26, -88.3985) -> (122.382, -88.2765)
  line L657 (122.382, -88.2765) -> (122.526, -88.1806)
  line L658 (122.526, -88.1806) -> (122.685, -88.1145)
  line L659 (135.428, -79.8181) -> (135.284, -79.914)
  line L660 (135.284, -79.914) -> (135.125, -79.9801)
  line L661 (135.125, -79.9801) -> (134.955, -80.0137)
  line L662 (136.225, -80.4609) -> (136.395, -80.4945)
  line L663 (135.125, -78.2948) -> (135.284, -78.3609)
  line L664 (135.284, -78.3609) -> (135.428, -78.4568)
  line L665 (122.164, -89.3722) -> (122.098, -89.2128)
  line L666 (122.098, -89.2128) -> (122.065, -89.0435)
  line L667 (122.065, -89.0435) -> (122.065, -88.8708)
  line L668 (134.454, -79.914) -> (134.311, -79.8181)
  line L669 (134.311, -79.8181) -> (134.188, -79.6961)
  line L670 (134.188, -79.6961) -> (134.093, -79.5525)
  line L671 (135.428, -78.4568) -> (135.55, -78.5788)
  line L672 (135.55, -78.5788) -> (135.646, -78.7224)
  line L673 (135.646, -78.7224) -> (135.712, -78.8818)
  line L674 (122.526, -89.7337) -> (122.382, -89.6378)
  line L675 (122.382, -89.6378) -> (122.26, -89.5158)
  line L676 (122.26, -89.5158) -> (122.164, -89.3722)
  line L677 (135.724, -80.5606) -> (135.884, -80.4945)
  line L678 (135.884, -80.4945) -> (136.053, -80.4609)
  line L679 (136.053, -80.4609) -> (136.225, -80.4609)
  line L680 (135.712, -78.8818) -> (135.745, -79.0511)
  line L681 (135.745, -79.0511) -> (135.745, -79.2238)
  line L682 (135.745, -79.2238) -> (135.712, -79.3931)
  line L683 (123.784, -88.7015) -> (123.817, -88.8708)
  line L684 (123.817, -88.8708) -> (123.817, -89.0435)
  line L685 (123.817, -89.0435) -> (123.784, -89.2128)
  line L686 (140.538, -90.6946) -> (140.443, -90.5511)
  line L687 (140.443, -90.5511) -> (140.376, -90.3916)
  line L688 (140.376, -90.3916) -> (140.343, -90.2223)
  line L689 (141.305, -89.2597) -> (141.475, -89.2933)
  line L690 (123.196, -88.1145) -> (123.356, -88.1806)
  line L691 (123.356, -88.1806) -> (123.499, -88.2765)
  line L692 (140.964, -90.9786) -> (140.804, -90.9125)
  line L693 (140.804, -90.9125) -> (140.661, -90.8166)
  line L694 (140.661, -90.8166) -> (140.538, -90.6946)
  line L695 (140.343, -90.2223) -> (140.343, -90.0497)
  line L696 (140.343, -90.0497) -> (140.376, -89.8804)
  line L697 (140.376, -89.8804) -> (140.443, -89.7209)
  line L698 (142.095, -90.2223) -> (142.062, -90.3916)
  line L699 (142.062, -90.3916) -> (141.996, -90.5511)
  line L700 (141.996, -90.5511) -> (141.9, -90.6946)
  line L701 (123.027, -89.8335) -> (122.855, -89.8335)
  line L702 (122.855, -89.8335) -> (122.685, -89.7998)
  line L703 (122.685, -89.7998) -> (122.526, -89.7337)
  line L704 (123.499, -88.2765) -> (123.622, -88.3985)
  line L705 (123.622, -88.3985) -> (123.717, -88.5421)
  line L706 (123.717, -88.5421) -> (123.784, -88.7015)
  line L707 (141.9, -90.6946) -> (141.778, -90.8166)
  line L708 (141.778, -90.8166) -> (141.634, -90.9125)
  line L709 (141.634, -90.9125) -> (141.475, -90.9786)
  line L710 (140.804, -89.3594) -> (140.964, -89.2933)
  line L711 (140.964, -89.2933) -> (141.133, -89.2597)
  line L712 (141.133, -89.2597) -> (141.305, -89.2597)
  line L713 (123.784, -89.2128) -> (123.717, -89.3722)
  line L714 (123.717, -89.3722) -> (123.622, -89.5158)
  line L715 (123.622, -89.5158) -> (123.499, -89.6378)
  line L716 (123.499, -89.6378) -> (123.356, -89.7337)
  line L717 (123.356, -89.7337) -> (123.196, -89.7998)
  line L718 (123.196, -89.7998) -> (123.027, -89.8335)
  line L719 (122.065, -88.8708) -> (122.098, -88.7015)
  line L720 (122.098, -88.7015) -> (122.164, -88.5421)
  line L721 (122.164, -88.5421) -> (122.26, -88.3985)
  line L722 (122.685, -88.1145) -> (122.855, -88.0809)
  line L723 (122.855, -88.0809) -> (123.027, -88.0809)
  line L724 (123.027, -88.0809) -> (123.196, -88.1145)
  line L725 (140.205, -87.0936) -> (140.364, -87.1597)
  line L726 (140.364, -87.1597) -> (140.508, -87.2556)
  line L727 (140.508, -87.2556) -> (140.63, -87.3777)
  line L728 (140.63, -87.3777) -> (140.726, -87.5212)
  line L729 (140.726, -87.5212) -> (140.792, -87.6807)
  line L730 (140.792, -87.6807) -> (140.825, -87.85)
  line L731 (141.475, -90.9786) -> (141.305, -91.0123)
  line L732 (141.305, -91.0123) -> (141.133, -91.0123)
  line L733 (141.133, -91.0123) -> (140.964, -90.9786)
  line L734 (140.825, -87.85) -> (140.825, -88.0226)
  line L735 (140.825, -88.0226) -> (140.792, -88.1919)
  line L736 (140.792, -88.1919) -> (140.726, -88.3513)
  line L737 (125.736, -92.5139) -> (125.896, -92.58)
  line L738 (125.896, -92.58) -> (126.039, -92.6759)
  line L739 (126.039, -92.6759) -> (126.162, -92.798)
  line L740 (133.659, -105.874) -> (133.782, -105.996)
  line L741 (128.206, -115.392) -> (128.074, -115.711)
  line L742 (128.074, -115.711) -> (127.882, -115.998)
  line L743 (127.882, -115.998) -> (127.639, -116.241)
  line L744 (137.828, -91.9614) -> (137.669, -92.0274)
  line L745 (137.669, -92.0274) -> (137.5, -92.061)
  line L746 (144.549, -85.852) -> (144.249, -85.852)
  line L747 (144.249, -85.852) -> (143.954, -85.7934)
  line L748 (143.954, -85.7934) -> (143.677, -85.6786)
  line L749 (137.5, -92.061) -> (137.328, -92.061)
  line L750 (137.328, -92.061) -> (137.159, -92.0274)
  line L751 (137.159, -92.0274) -> (137, -91.9614)
  line L752 (137, -91.9614) -> (136.856, -91.8657)
  line L753 (123.652, -91.8375) -> (123.53, -91.7155)
  line L754 (123.53, -91.7155) -> (123.434, -91.5719)
  line L755 (123.434, -91.5719) -> (123.368, -91.4125)
  line L756 (137.577, -104.202) -> (137.653, -104.316)
  line L757 (137.653, -104.316) -> (137.706, -104.444)
  line L758 (137.706, -104.444) -> (137.733, -104.579)
  line L759 (143.048, -85.0499) -> (142.934, -84.7725)
  line L760 (142.934, -84.7725) -> (142.875, -84.4781)
  line L761 (142.875, -84.4781) -> (142.875, -84.1779)
  line L762 (142.875, -84.1779) -> (142.934, -83.8835)
  line L763 (142.934, -83.8835) -> (143.048, -83.6061)
  line L764 (143.048, -83.6061) -> (143.215, -83.3565)
  line L765 (138.09, -82.9782) -> (138.186, -83.1218)
  line L766 (138.186, -83.1218) -> (138.252, -83.2812)
  line L767 (138.252, -83.2812) -> (138.285, -83.4505)
  line L768 (123.368, -91.4125) -> (123.335, -91.2432)
  line L769 (123.335, -91.2432) -> (123.335, -91.0705)
  line L770 (123.335, -91.0705) -> (123.368, -90.9012)
  line L771 (145.905, -96.8214) -> (145.872, -96.9907)
  line L772 (145.872, -96.9907) -> (145.806, -97.1502)
  line L773 (145.806, -97.1502) -> (145.71, -97.2937)
  line L774 (149.52, -103.893) -> (149.398, -104.015)
  line L775 (149.398, -104.015) -> (149.254, -104.111)
  line L776 (149.254, -104.111) -> (149.095, -104.177)
  line L777 (149.095, -104.177) -> (148.925, -104.21)
  line L778 (137.665, -82.6942) -> (137.824, -82.7603)
  line L779 (137.824, -82.7603) -> (137.968, -82.8562)
  line L780 (137.968, -82.8562) -> (138.09, -82.9782)
  line L781 (132.324, -106.97) -> (132.258, -106.81)
  line L782 (132.258, -106.81) -> (132.225, -106.641)
  line L783 (132.225, -106.641) -> (132.225, -106.468)
  line L784 (146.714, -98.1582) -> (146.858, -98.2541)
  line L785 (146.858, -98.2541) -> (146.98, -98.3762)
  line L786 (145.71, -96.1765) -> (145.806, -96.32)
  line L787 (134.457, -107.878) -> (134.626, -107.912)
  line L788 (133.356, -105.712) -> (133.516, -105.778)
  line L789 (133.516, -105.778) -> (133.659, -105.874)
  line L790 (132.542, -105.874) -> (132.686, -105.778)
  line L791 (132.686, -105.778) -> (132.845, -105.712)
  line L792 (132.845, -105.712) -> (133.015, -105.678)
  line L793 (126.013, -116.565) -> (125.694, -116.433)
  line L794 (125.694, -116.433) -> (125.407, -116.241)
  line L795 (125.407, -116.241) -> (125.164, -115.998)
  line L796 (127.033, -116.565) -> (126.695, -116.632)
  line L797 (126.695, -116.632) -> (126.351, -116.632)
  line L798 (126.351, -116.632) -> (126.013, -116.565)
  line L799 (143.954, -82.8626) -> (144.249, -82.804)
  line L800 (144.249, -82.804) -> (144.549, -82.804)
  line L801 (144.549, -82.804) -> (144.844, -82.8626)
  line L802 (145.71, -97.2937) -> (145.588, -97.4158)
  line L803 (145.588, -97.4158) -> (145.444, -97.5117)
  line L804 (145.444, -97.5117) -> (145.285, -97.5777)
  line L805 (145.285, -97.5777) -> (145.115, -97.6114)
  line L806 (133.015, -107.431) -> (132.845, -107.397)
  line L807 (132.845, -107.397) -> (132.686, -107.331)
  line L808 (132.686, -107.331) -> (132.542, -107.235)
  line L809 (133.956, -107.978) -> (134.115, -107.912)
  line L810 (134.115, -107.912) -> (134.285, -107.878)
  line L811 (134.285, -107.878) -> (134.457, -107.878)
  line L812 (123.368, -90.9012) -> (123.434, -90.7418)
  line L813 (123.434, -90.7418) -> (123.53, -90.5982)
  line L814 (123.53, -90.5982) -> (123.652, -90.4762)
  line L815 (133.659, -107.235) -> (133.516, -107.331)
  line L816 (133.516, -107.331) -> (133.356, -107.397)
  line L817 (133.356, -107.397) -> (133.187, -107.431)
  line L818 (124.125, -90.2806) -> (124.297, -90.2806)
  line L819 (124.297, -90.2806) -> (124.466, -90.3142)
  line L820 (141.475, -89.2933) -> (141.634, -89.3594)
  line L821 (123.652, -90.4762) -> (123.796, -90.3803)
  line L822 (123.796, -90.3803) -> (123.955, -90.3142)
  line L823 (123.955, -90.3142) -> (124.125, -90.2806)
  line L824 (143.215, -83.3565) -> (143.428, -83.1442)
  line L825 (143.428, -83.1442) -> (143.677, -82.9774)
  line L826 (143.677, -82.9774) -> (143.954, -82.8626)
  line L827 (132.225, -106.468) -> (132.258, -106.299)
  line L828 (132.258, -106.299) -> (132.324, -106.14)
  line L829 (132.324, -106.14) -> (132.42, -105.996)
  line L830 (146.98, -98.3762) -> (147.076, -98.5197)
  line L831 (147.076, -98.5197) -> (147.142, -98.6792)
  line L832 (147.142, -98.6792) -> (147.175, -98.8485)
  line L833 (147.175, -98.8485) -> (147.175, -99.0211)
  line L834 (147.175, -99.0211) -> (147.142, -99.1904)
  line L835 (133.977, -106.468) -> (133.977, -106.641)
  line L836 (133.977, -106.641) -> (133.944, -106.81)
  line L837 (138.255, -90.9308) -> (138.289, -91.0998)
  line L838 (138.289, -91.0998) -> (138.289, -91.2722)
  line L839 (138.289, -91.2722) -> (138.255, -91.4412)
  line L840 (138.255, -91.4412) -> (138.189, -91.6005)
  line L841 (138.189, -91.6005) -> (138.094, -91.7438)
  line L842 (143.677, -85.6786) -> (143.428, -85.5118)
  line L843 (143.428, -85.5118) -> (143.215, -85.2995)
  line L844 (143.215, -85.2995) -> (143.048, -85.0499)
  line L845 (137.61, -94.2721) -> (137.996, -94.3487)
  line L846 (145.285, -95.8925) -> (145.444, -95.9585)
  line L847 (145.444, -95.9585) -> (145.588, -96.0544)
  line L848 (145.588, -96.0544) -> (145.71, -96.1765)
  line L849 (143.201, -93.8547) -> (143.344, -93.7588)
  line L850 (143.344, -93.7588) -> (143.504, -93.6928)
  line L851 (143.504, -93.6928) -> (143.673, -93.6591)
  line L852 (147.154, -100.358) -> (147.314, -100.292)
  line L853 (147.314, -100.292) -> (147.483, -100.258)
  line L854 (145.115, -97.6114) -> (144.943, -97.6114)
  line L855 (133.69, -108.196) -> (133.812, -108.074)
  line L856 (133.812, -108.074) -> (133.956, -107.978)
  line L857 (138.186, -83.9519) -> (138.09, -84.0955)
  line L858 (138.09, -84.0955) -> (137.968, -84.2175)
  line L859 (137.968, -84.2175) -> (137.824, -84.3134)
  line L860 (133.782, -105.996) -> (133.877, -106.14)
  line L861 (133.877, -106.14) -> (133.944, -106.299)
  line L862 (133.944, -106.299) -> (133.977, -106.468)
  line L863 (133.015, -105.678) -> (133.187, -105.678)
  line L864 (133.187, -105.678) -> (133.356, -105.712)
  line L865 (132.42, -105.996) -> (132.542, -105.874)
  line L866 (143.673, -93.6591) -> (143.845, -93.6591)
  line L867 (143.845, -93.6591) -> (144.015, -93.6928)
  line L868 (133.187, -107.431) -> (133.015, -107.431)
  line L869 (138.285, -83.4505) -> (138.285, -83.6232)
  line L870 (138.285, -83.6232) -> (138.252, -83.7925)
  line L871 (138.252, -83.7925) -> (138.186, -83.9519)
  line L872 (145.806, -96.32) -> (145.872, -96.4795)
  line L873 (145.872, -96.4795) -> (145.905, -96.6488)
  line L874 (145.905, -96.6488) -> (145.905, -96.8214)
  line L875 (145.37, -85.5118) -> (145.121, -85.6786)
  line L876 (145.121, -85.6786) -> (144.844, -85.7934)
  line L877 (144.844, -85.7934) -> (144.549, -85.852)
  line L878 (133.944, -106.81) -> (133.877, -106.97)
  line L879 (133.877, -106.97) -> (133.782, -107.113)
  line L880 (133.782, -107.113) -> (133.659, -107.235)
  line L881 (137.237, -103.975) -> (137.365, -104.028)
  line L882 (137.365, -104.028) -> (137.479, -104.104)
  line L883 (137.479, -104.104) -> (137.577, -104.202)
  line L884 (132.542, -107.235) -> (132.42, -107.113)
  line L885 (132.42, -107.113) -> (132.324, -106.97)
  line L886 (127.639, -116.241) -> (127.352, -116.433)
  line L887 (127.352, -116.433) -> (127.033, -116.565)
  line L888 (138.094, -91.7438) -> (137.972, -91.8657)
  line L889 (137.972, -91.8657) -> (137.828, -91.9614)
  line L890 (149.616, -103.749) -> (149.52, -103.893)
  line L891 (148.531, -116.672) -> (148.193, -116.605)
  line L892 (150.453, -115.094) -> (150.386, -115.432)
  line L893 (145.864, -84.7725) -> (145.75, -85.0499)
  line L894 (145.75, -85.0499) -> (145.583, -85.2995)
  line L895 (145.583, -85.2995) -> (145.37, -85.5118)
  line L896 (144.153, -96.6488) -> (144.186, -96.4795)
  line L897 (144.186, -96.4795) -> (144.253, -96.32)
  line L898 (144.253, -96.32) -> (144.348, -96.1765)
  line L899 (144.348, -96.1765) -> (144.471, -96.0544)
  line L900 (148.591, -79.642) -> (148.253, -79.5747)
  line L901 (148.253, -79.5747) -> (147.934, -79.4428)
  line L902 (147.934, -79.4428) -> (147.647, -79.2513)
  line L903 (149.095, -102.492) -> (149.254, -102.558)
  line L904 (149.254, -102.558) -> (149.398, -102.654)
  line L905 (149.398, -102.654) -> (149.52, -102.776)
  line L906 (149.52, -102.776) -> (149.616, -102.919)
  line L907 (120.364, -93.8112) -> (120.683, -93.6793)
  line L908 (120.683, -93.6793) -> (121.021, -93.612)